Autodesk Fusion 360 part; units mm, degrees
note: some values were not read from the file. Set by a fixed rule: which sketch regions a step uses.
(part 2 of 2)
  line L769 (-18.5, 34.5566) -> (-18.5, 37.4434)
  line L770 (-21, 33.1132) -> (-18.5, 34.5566)
  line L771 (-23.5, 34.5566) -> (-21, 33.1132)
  line L772 (-23.5, 37.4434) -> (-23.5, 34.5566)
  line L773 (3.5, 39.1754) -> (6, 40.6188)
  line L774 (6, 40.6188) -> (6, 43.5056)
  line L775 (6, 43.5056) -> (3.5, 44.9489)
  line L776 (3.5, 44.9489) -> (1, 43.5056)
  line L777 (1, 43.5056) -> (1, 40.6188)
  line L778 (1, 40.6188) -> (3.5, 39.1754)
  line L779 (2.5, 37.4434) -> (0, 38.8868)
  line L780 (2.5, 34.5566) -> (2.5, 37.4434)
  line L781 (0, 33.1132) -> (2.5, 34.5566)
  line L782 (-2.5, 34.5566) -> (0, 33.1132)
  line L783 (-2.5, 37.4434) -> (-2.5, 34.5566)
  line L784 (0, 38.8868) -> (-2.5, 37.4434)
  line L785 (-3.5, 39.1754) -> (-1, 40.6188)
  line L786 (-1, 40.6188) -> (-1, 43.5056)
  line L787 (-1, 43.5056) -> (-3.5, 44.9489)
  line L788 (-6, 40.6188) -> (-3.5, 39.1754)
  line L789 (-3.5, 44.9489) -> (-6, 43.5056)
  line L790 (-6, 43.5056) -> (-6, 40.6188)
  line L791 (-7, 38.8868) -> (-9.5, 37.4434)
  line L792 (-4.5, 37.4434) -> (-7, 38.8868)
  line L793 (-4.5, 34.5566) -> (-4.5, 37.4434)
  line L794 (-7, 33.1132) -> (-4.5, 34.5566)
  line L795 (-9.5, 34.5566) -> (-7, 33.1132)
  line L796 (-9.5, 37.4434) -> (-9.5, 34.5566)
  line L797 (17.5, 39.1754) -> (20, 40.6188)
  line L798 (20, 40.6188) -> (20, 43.5056)
  line L799 (20, 43.5056) -> (17.5, 44.9489)
  line L800 (17.5, 44.9489) -> (15, 43.5056)
  line L801 (15, 43.5056) -> (15, 40.6188)
  line L802 (15, 40.6188) -> (17.5, 39.1754)
  line L803 (16.5, 37.4434) -> (14, 38.8868)
  line L804 (16.5, 34.5566) -> (16.5, 37.4434)
  line L805 (14, 33.1132) -> (16.5, 34.5566)
  line L806 (11.5, 34.5566) -> (14, 33.1132)
  line L807 (11.5, 37.4434) -> (11.5, 34.5566)
  line L808 (14, 38.8868) -> (11.5, 37.4434)
  line L809 (10.5, 39.1754) -> (13, 40.6188)
  line L810 (13, 40.6188) -> (13, 43.5056)
  line L811 (13, 43.5056) -> (10.5, 44.9489)
  line L812 (8, 40.6188) -> (10.5, 39.1754)
  line L813 (10.5, 44.9489) -> (8, 43.5056)
  line L814 (8, 43.5056) -> (8, 40.6188)
  line L815 (7, 38.8868) -> (4.5, 37.4434)
  line L816 (9.5, 37.4434) -> (7, 38.8868)
  line L817 (9.5, 34.5566) -> (9.5, 37.4434)
  line L818 (7, 33.1132) -> (9.5, 34.5566)
  line L819 (4.5, 34.5566) -> (7, 33.1132)
  line L820 (4.5, 37.4434) -> (4.5, 34.5566)
  line L821 (31.5, 39.1754) -> (34, 40.6188)
  line L822 (34, 40.6188) -> (34, 43.5056)
  line L823 (34, 43.5056) -> (31.5, 44.9489)
  line L824 (31.5, 44.9489) -> (29, 43.5056)
  line L825 (29, 43.5056) -> (29, 40.6188)
  line L826 (29, 40.6188) -> (31.5, 39.1754)
  line L827 (30.5, 37.4434) -> (28, 38.8868)
  line L828 (30.5, 34.5566) -> (30.5, 37.4434)
  line L829 (28, 33.1132) -> (30.5, 34.5566)
  line L830 (25.5, 34.5566) -> (28, 33.1132)
  line L831 (25.5, 37.4434) -> (25.5, 34.5566)
  line L832 (28, 38.8868) -> (25.5, 37.4434)
  line L833 (24.5, 39.1754) -> (27, 40.6188)
  line L834 (27, 40.6188) -> (27, 43.5056)
  line L835 (27, 43.5056) -> (24.5, 44.9489)
  line L836 (22, 40.6188) -> (24.5, 39.1754)
  line L837 (24.5, 44.9489) -> (22, 43.5056)
  line L838 (22, 43.5056) -> (22, 40.6188)
  line L839 (21, 38.8868) -> (18.5, 37.4434)
  line L840 (23.5, 37.4434) -> (21, 38.8868)
  line L841 (23.5, 34.5566) -> (23.5, 37.4434)
  line L842 (21, 33.1132) -> (23.5, 34.5566)
  line L843 (18.5, 34.5566) -> (21, 33.1132)
  line L844 (18.5, 37.4434) -> (18.5, 34.5566)
  line L845 (25, 31.5) -> (-25, 31.5)
  line L846 (-25, -31.5) -> (25, -31.5)
  point P0 (-3.5, 6.0622)
  point P1 (-7, 0)
  point P2 (3.5, 6.0622)
  dimension "d440" = 5
  dimension "d441" = 2
  dimension "d444" = 14
  dimension "d445" = 12
  constraint equal L6 L9
  constraint parallel L6 L9
  constraint vertical L7
  constraint perpendicular L6 L14
  constraint parallel L7 L19
  constraint equal L7 L19
  constraint horizontal L2.start L18.end
  constraint perpendicular L8 L21
  constraint equal L5 L23
  constraint parallel L5 L23
  constraint horizontal L9.end L22.end
  constraint perpendicular L5 L28
  measures "d440" distance of L4 L7
  measures "d441" distance of L6 L9
extrude "Extrusion7" cut sketch "Skizze9" against normal up to surface (2 mm away) contours L101 L102 L103 L104 L105 L106 L846 | L113 L114 L115 L116 L117 L118 L846 | L77 L78 L79 L80 L81 L82 L846 | L89 L90 L91 L92 L93 L94 L846 | L53 L54 L55 L56 L57 L58 L846 | L65 L66 L67 L68 L69 L70 L846 | L677 L678 L681 L682 L845 | L689 L690 L692 L694 L845 | L653 L654 L657 L658 L845 | L665 L666 L668 L670 L845 | L629 L630 L633 L634 L845 | L641 L642 L644 L646 L845 | L2 L3 L4 L5 L6 L7 | L8 L9 L10 L11 L12 L13 | L15 L16 L17 L18 L19 L20 | L22 L23 L24 L25 L26 L27 | L173 L174 L175 L176 L177 L178 | L179 L180 L181 L182 L183 L184 | L185 L186 L187 L188 L189 L190 | L197 L198 L199 L200 L201 L202 | L203 L204 L205 L206 L207 L208 | L209 L210 L211 L212 L213 L214 | L215 L216 L217 L218 L219 L220 | L221 L222 L223 L224 L225 L226 | L227 L228 L229 L230 L231 L232 | L233 L234 L235 L236 L237 L238 | L239 L240 L241 L242 L243 L244 | L293 L294 L295 L296 L297 L298 | L299 L300 L301 L302 L303 L304 | L305 L306 L307 L308 L309 L310 | L317 L318 L319 L320 L321 L322 | L323 L324 L325 L326 L327 L328 | L329 L330 L331 L332 L333 L334 | L335 L336 L337 L338 L339 L340 | L341 L342 L343 L344 L345 L346 | L347 L348 L349 L350 L351 L352 | L353 L354 L355 L356 L357 L358 | L359 L360 L361 L362 L363 L364 | L413 L414 L415 L416 L417 L418 | L419 L420 L421 L422 L423 L424 | L425 L426 L427 L428 L429 L430 | L437 L438 L439 L440 L441 L442 | L443 L444 L445 L446 L447 L448 | L449 L450 L451 L452 L453 L454 | L455 L456 L457 L458 L459 L460 | L509 L510 L511 L512 L513 L514 | L515 L516 L517 L518 L519 L520 | L521 L522 L523 L524 L525 L526 | L533 L534 L535 L536 L537 L538 | L539 L540 L541 L542 L543 L544 | L545 L546 L547 L548 L549 L550 | L551 L552 L553 L554 L555 L556 | L557 L558 L559 L560 L561 L562 | L563 L564 L565 L566 L567 L568 | L569 L570 L571 L572 L573 L574 | L575 L576 L577 L578 L579 L580 | L635 L636 L637 L638 L639 L640 | L659 L660 L661 L662 L663 L664 | L671 L672 L673 L674 L675 L676 | L683 L684 L685 L686 L687 L688 | L695 L696 L697 L698 L699 L700
equation "d357 = 93 mm + 2 * 2 mm"
equation "d371 = 25 mm + ( 2 * 0.5 ) * 1 mm"
equation "d372 = d371 / 2"
equation "d408 = d407 / 2"
named bodies: "Door_Mount"
